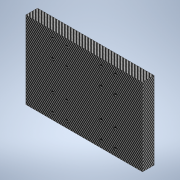
# Autodesk Inventor part: Placa5 Base Extrusor
Saved by Autodesk Inventor 2022 (Build 260153000, 153)
## iProperties
Created: 2021-11-08
Part Number: Placa5 Base Extrusor
Material: CFRP
Document SubType Name: Modeling
Designer: Samuel Gómez
Density: 1.43 g/cm^3
Appearance: Carbon Fiber
Author: Samuel Gómez
Autodesk Inventor part; units mm, degrees
ref_plane "YZ Plane" through (0, 0, 0) normal (1, 0, 0) x (0, 1, 0)
ref_plane "XZ Plane" through (0, 0, 0) normal (0, 1, 0) x (-1, 0, 0)
ref_plane "XY Plane" through (0, 0, 0) normal (0, 0, 1) x (1, 0, 0)
sketch "Boceto1" plane through (0, 0, 0) normal (0, 0, 1) x (1, 0, 0)
  line L0 (0, 0) -> (150, 0)
  line L1 (150, 0) -> (150, 100)
  line L2 (150, 100) -> (0, 100)
  line L3 (0, 100) -> (0, 0)
  dimension "d0" = 150
  dimension "d1" = 100
  constraints: 8 end point, 2 parallel, 1 horizontal, 1 perpendicular
  measures "d0" distance of L1.end L2.end
  measures "d1" distance of L2.end L0.start
extrude "Extrusión1" add sketch "Boceto1" along normal blind 15
sketch "Boceto2" plane through (0, 0, 15) normal (0, 0, 1) x (1, 0, 0)
  line L0 (0, 100) -> (0, 0) projected
  line L1 (0, 50) -> (150, 50) construction
  line L2 (150, 0) -> (150, 100) projected
  line L3 (35, 50) -> (35, 8.625) construction
  line L4 (35, 31.375) -> (53.4, 31.375) construction
  circle A0 centre (35, 8.625) radius 1.75
  circle A1 centre (35, 31.375) radius 1.75
  circle A2 centre (53.4, 31.375) radius 1.75
  line L5 (35, 8.625) -> (53.4, 8.625) construction
  line L6 (53.4, 8.625) -> (53.4, 31.375) construction
  circle A3 centre (53.4, 8.625) radius 1.75
  line L7 (75, 50) -> (75, -45.8992) construction
  line L8 (115, 31.375) -> (96.6, 31.375) construction
  circle A4 centre (115, 8.625) radius 1.75
  circle A5 centre (115, 31.375) radius 1.75
  circle A6 centre (96.6, 31.375) radius 1.75
  line L9 (115, 8.625) -> (96.6, 8.625) construction
  line L10 (96.6, 8.625) -> (96.6, 31.375) construction
  circle A7 centre (96.6, 8.625) radius 1.75
  line L11 (35, 68.625) -> (53.4, 68.625) construction
  circle A8 centre (35, 91.375) radius 1.75
  circle A9 centre (35, 68.625) radius 1.75
  circle A10 centre (53.4, 68.625) radius 1.75
  line L12 (35, 91.375) -> (53.4, 91.375) construction
  line L13 (53.4, 91.375) -> (53.4, 68.625) construction
  circle A11 centre (53.4, 91.375) radius 1.75
  circle A12 centre (115, 68.625) radius 1.75
  circle A13 centre (115, 91.375) radius 1.75
  line L14 (115, 68.625) -> (96.6, 68.625) construction
  circle A14 centre (96.6, 68.625) radius 1.75
  line L15 (115, 91.375) -> (96.6, 91.375) construction
  line L16 (96.6, 91.375) -> (96.6, 68.625) construction
  circle A15 centre (96.6, 91.375) radius 1.75
  dimension "d4" = 41.375
  dimension "d5" = 18.625
  dimension "d6" = 18.4
  dimension "d7" = 3.5
  dimension "d8" = 3.5
  dimension "d9" = 3.5
  dimension "d10" = 3.5
  dimension "d13" = 40
  constraints: 30 end point, 24 symmetric about line, 16 centre point, 16 coincident, 3 midpoint, 3 perpendicular, 2 point on line, 1 horizontal, 1 vertical, 12 other
  measures "d4" distance of L3.start L3.end
  measures "d5" distance from line of L4.end L1
  measures "d6" distance of L4.start L4.end
  measures "d7" diameter of A0
  measures "d8" diameter of A1
  measures "d9" diameter of A2
  measures "d10" diameter of A3
  measures "d13" distance between parallel lines of L7 L3
extrude "Extrusión2" cut sketch "Boceto2" against normal up to surface (15 mm away)
